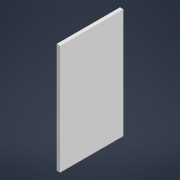
# Autodesk Inventor part: N_into_side
Saved by Autodesk Inventor 2022 (Build 260153070, 153G)
## iProperties
Created: 2021-11-16
Part Number: N_into_side
Material: Типовые
Document SubType Name: Modeling
Designer: kalugin_a
Density: 1 g/cm^3
Appearance: По умолчанию
Author: kalugin_a
Autodesk Inventor part; units mm, degrees
ref_plane "YZ Plane" through (0, 0, 0) normal (1, 0, 0) x (0, 1, 0)
ref_plane "XZ Plane" through (0, 0, 0) normal (0, 1, 0) x (-1, 0, 0)
ref_plane "XY Plane" through (0, 0, 0) normal (0, 0, 1) x (1, 0, 0)
sketch "Эскиз2" plane through (0, 0, 0) normal (1, 0, 0) x (0, 1, 0)
  line L0 (-139, -2) -> (381, -2)
  line L1 (381, -2) -> (381, -302)
  line L2 (381, -302) -> (-139, -302)
  line L3 (-139, -302) -> (-139, -2)
  dimension "d0" = 300
  dimension "d4" = 520
  constraints: 8 end point, 1 horizontal, 1 parallel
  measures "d0" distance of L0.end L1.end
  measures "d4" distance of L1.end L2.end
extrude "Выдавливание1" add sketch "Эскиз2" along normal blind 16
